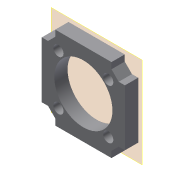
# Autodesk Inventor part: 50_Cube_Insert_Thorlabs
Saved by Autodesk Inventor 2019.4 (Build 234330000, 330)
## iProperties
Created: 2019-07-01
Part Number: 50_Cube_Insert_Thorlabs
Material: Generic
Document SubType Name: Modeling
Designer: diederichbenedict
Density: 1 g/cm^3
Appearance: Default
Author: diederichbenedict
Autodesk Inventor part; units mm, degrees
ref_plane "YZ Plane" through (0, 0, 0) normal (1, 0, 0) x (0, 1, 0)
ref_plane "XZ Plane" through (0, 0, 0) normal (0, 1, 0) x (-1, 0, 0)
ref_plane "Work Plane1" through (0, 0, 10) normal (0, 0, 1) x (1, 0, 0)
sketch "Sketch1" plane through (0, 0, 10) normal (0, 0, 1) x (1, 0, 0)
  line L0 (-4.0299, -0.3538) -> (-2.2322, 1.4439) construction
  arc A0 (-1.4439, 2.2322) -> (-2.2322, 1.4439) centre (-0.9299, 0.9299) ccw construction
  line L1 (-1.4439, 2.2322) -> (0.3538, 4.0299) construction
  line L2 (-37.8299, 42.8299) -> (-37.8299, 37.8299) construction
  line L3 (-37.8299, 37.8299) -> (-42.9208, 37.8299) construction
  line L4 (-37.8299, 42.2137) -> (-37.8299, 45.8299) construction
  line L5 (-37.8299, 45.8299) -> (-4.0299, 45.8299) construction
  line L6 (-4.0299, 45.8299) -> (-4.0299, 42.2137) construction
  line L7 (-4.0299, 4.0299) -> (0.3538, 4.0299) projected
  circle A1 centre (-20.9299, 20.9299) radius 17.5 projected
  line L8 (-20.9299, 58.9723) -> (17.1124, 20.9299) construction
  line L9 (17.1124, 20.9299) -> (-20.9299, -17.1124) construction
  line L10 (-20.9299, -17.1124) -> (-58.9723, 20.9299) construction
  line L11 (-58.9723, 20.9299) -> (-20.9299, 58.9723) construction
  line L12 (-20.9299, 58.9723) -> (-20.9299, -17.1124) construction
  line L13 (17.1124, 20.9299) -> (-58.9723, 20.9299) construction
  line L14 (-20.9299, 58.9723) -> (32.8701, 58.9723) construction
  line L15 (-43.4299, 43.4299) -> (1.5701, 43.4299) construction
  line L16 (1.5701, 43.4299) -> (1.5701, -1.5701) construction
  line L17 (1.5701, -1.5701) -> (-43.4299, -1.5701) construction
  line L18 (-43.4299, -1.5701) -> (-43.4299, 43.4299) construction
  line L19 (-43.4299, 43.4299) -> (1.5701, -1.5701) construction
  line L20 (1.5701, 43.4299) -> (-43.4299, -1.5701) construction
  line L21 (-43.4299, 5.3876) -> (-43.4299, 36.4723)
  line L22 (-43.4299, 36.4723) -> (-36.4723, 43.4299)
  line L23 (-36.4723, 43.4299) -> (-5.3876, 43.4299)
  line L24 (-5.3876, 43.4299) -> (1.5701, 36.4723)
  line L25 (1.5701, 36.4723) -> (1.5701, 5.3876)
  line L26 (1.5701, 5.3876) -> (-5.3876, -1.5701)
  line L27 (-5.3876, -1.5701) -> (-36.4723, -1.5701)
  line L28 (-36.4723, -1.5701) -> (-43.4299, 5.3876)
  line L29 (-4.0299, 42.2137) -> (-37.8299, 42.2137) projected
  line L30 (-4.0299, -0.3538) -> (-4.0299, 4.0299) projected
  point P0 (-37.8299, 4.0299)
  point P1 (-20.9299, 20.9299)
  dimension "d18" = 53.8
  dimension "d19" = 45
  dimension "d20" = 53.8
  dimension "d21" = 45
  dimension "d22" = 45
  constraints: 42 end point, 15 point on line, 5 midpoint, 4 parallel, 3 perpendicular, 2 horizontal, 1 equal length
  measures "d18" distance of L8.start L8.end
  measures "d19" angle of L8 L14
  measures "d20" distance of L8.end L9.end
  measures "d21" distance of L16.end L17.end
  measures "d22" distance of L15.end L16.end
extrude "Extrusion1" add sketch "Sketch1" along normal blind 8
sketch "Sketch2" plane through (0, 0, 18) normal (0, 0, 1) x (1, 0, 0)
  circle A0 centre (-35.9299, 35.9299) radius 3.0099 construction
  circle A1 centre (-5.93, 35.9299) radius 3.0099 construction
  circle A2 centre (-5.93, 5.93) radius 3.0099 construction
  circle A3 centre (-35.9299, 5.93) radius 3.0099 construction
  circle A4 centre (-35.9299, 35.9299) radius 3.05
  circle A5 centre (-5.93, 35.9299) radius 3.05
  circle A6 centre (-5.93, 5.93) radius 3.05
  circle A7 centre (-35.9299, 5.93) radius 3.05
  point P0 (0, 0)
  dimension "d30" = 6.1
  dimension "d31" = 6.1
  dimension "d32" = 6.1
  dimension "d33" = 6.1
  constraints: 4 centre point
  measures "d30" diameter of A4
  measures "d31" diameter of A5
  measures "d32" diameter of A6
  measures "d33" diameter of A7
ref_plane "Work Plane2" through (-40.9959, 0.8639, 22.2359) normal (0, 0, 1) x (1, 0, 0)
extrude "Extrusion2" cut sketch "Sketch2" against normal through all
sketch "Sketch3" plane through (0, 0, 10) normal (0, 0, -1) x (-1, 0, 0)
  line L0 (37.8299, -0.4701) -> (37.8299, 4.0299) construction
  line L1 (4.0299, 4.0299) -> (4.0299, -0.4701) construction
  line L2 (37.8299, -0.4701) -> (37.8299, 1.1886) construction
  line L3 (4.0299, -3.9701) -> (4.0299, -0.3538) construction
  line L4 (45.8299, 4.0299) -> (42.2137, 4.0299) construction
  line L5 (-0.3538, 4.0299) -> (-3.9701, 4.0299) construction
  line L6 (-3.9701, 37.8299) -> (-0.3538, 37.8299) construction
  line L7 (4.0299, 42.2137) -> (4.0299, 45.8299) construction
  line L8 (37.8299, 45.8299) -> (37.8299, 42.2137) construction
  line L9 (42.2137, 37.8299) -> (45.8299, 37.8299) construction
  line L10 (40.4657, 37.7299) -> (45.8299, 37.7299)
  line L11 (45.8299, 37.7299) -> (45.8299, 4.1299)
  line L12 (45.8299, 4.1299) -> (40.4657, 4.1299)
  line L13 (40.4657, 4.1299) -> (40.4657, 37.7299)
  line L14 (37.7299, 2.4952) -> (4.1299, 2.4952)
  line L15 (4.1299, 2.4952) -> (4.1299, -3.9701)
  line L16 (4.1299, -3.9701) -> (37.7299, -3.9701)
  line L17 (37.7299, -3.9701) -> (37.7299, 2.4952)
  line L18 (1.8946, 4.1299) -> (-3.9701, 4.1299)
  line L19 (-3.9701, 4.1299) -> (-3.9701, 37.7299)
  line L20 (-3.9701, 37.7299) -> (1.8946, 37.7299)
  line L21 (1.8946, 37.7299) -> (1.8946, 4.1299)
  line L22 (4.1299, 40.7326) -> (37.7299, 40.7326)
  line L23 (37.7299, 40.7326) -> (37.7299, 45.8299)
  line L24 (37.7299, 45.8299) -> (4.1299, 45.8299)
  line L25 (4.1299, 45.8299) -> (4.1299, 40.7326)
  point P0 (0, 0)
  dimension "d23" = 0.1
  dimension "d24" = 0.1
  dimension "d25" = 0.1
  dimension "d26" = 0.1
  dimension "d27" = 0.1
  constraints: 32 end point, 8 parallel, 4 horizontal, 4 perpendicular, 3 point on line
  measures "d23" distance between parallel lines of L8 L23
  measures "d24" distance between parallel lines of L7 L25
  measures "d25" distance between parallel lines of L6 L20
  measures "d26" distance between parallel lines of L5 L18
  measures "d27" distance between parallel lines of L1 L15
extrude "Extrusion3" add sketch "Sketch3" against normal up to surface (8 mm away)
sketch "Sketch4" plane through (0, 0, 18) normal (0, 0, 1) x (1, 0, 0)
  line L0 (3.9701, 4.1299) -> (0.3124, 4.1299) projected
  line L1 (3.9701, 37.7299) -> (3.9701, 4.1299) projected
  line L2 (0.3124, 37.7299) -> (3.9701, 37.7299) projected
  line L3 (0.3124, 37.7299) -> (-4.1299, 42.1723) projected
  line L4 (-4.1299, 45.8299) -> (-4.1299, 42.1723) projected
  line L5 (-37.7299, 45.8299) -> (-4.1299, 45.8299) projected
  line L6 (-37.7299, 42.1723) -> (-37.7299, 45.8299) projected
  line L7 (-37.7299, 42.1723) -> (-42.1723, 37.7299) projected
  line L8 (-45.8299, 37.7299) -> (-42.1723, 37.7299) projected
  line L9 (-45.8299, 4.1299) -> (-45.8299, 37.7299) projected
  line L10 (-42.1723, 4.1299) -> (-45.8299, 4.1299) projected
  line L11 (-42.1723, 4.1299) -> (-37.7299, -0.3124) projected
  line L12 (-37.7299, -3.9701) -> (-37.7299, -0.3124) projected
  line L13 (-4.1299, -3.9701) -> (-37.7299, -3.9701) projected
  line L14 (-4.1299, -0.3124) -> (-4.1299, -3.9701) projected
  line L15 (-4.1299, -0.3124) -> (0.3124, 4.1299) projected
  circle A0 centre (-20.9299, 20.9299) radius 17.5 projected
  circle A1 centre (-35.9299, 5.93) radius 3.05 projected
  circle A2 centre (-5.93, 35.9299) radius 3.05 projected
  circle A3 centre (-35.9299, 35.9299) radius 3.05 projected
  circle A4 centre (-5.93, 5.93) radius 3.05 projected
  line L16 (-3.9799, 45.9799) -> (-3.9799, 42.2344)
  line L17 (-3.9799, 42.2344) -> (0.3745, 37.8799)
  line L18 (0.3745, 37.8799) -> (4.1201, 37.8799)
  line L19 (4.1201, 37.8799) -> (4.1201, 3.9799)
  line L20 (4.1201, 3.9799) -> (0.3745, 3.9799)
  line L21 (0.3745, 3.9799) -> (-3.9799, -0.3745)
  line L22 (-3.9799, -0.3745) -> (-3.9799, -4.1201)
  line L23 (-3.9799, -4.1201) -> (-37.8799, -4.1201)
  line L24 (-37.8799, -4.1201) -> (-37.8799, -0.3745)
  line L25 (-37.8799, -0.3745) -> (-42.2344, 3.9799)
  line L26 (-42.2344, 3.9799) -> (-45.9799, 3.9799)
  line L27 (-45.9799, 3.9799) -> (-45.9799, 37.8799)
  line L28 (-45.9799, 37.8799) -> (-42.2344, 37.8799)
  line L29 (-42.2344, 37.8799) -> (-37.8799, 42.2344)
  line L30 (-37.8799, 42.2344) -> (-37.8799, 45.9799)
  line L31 (-37.8799, 45.9799) -> (-3.9799, 45.9799)
  point P0 (0, 0)
  dimension "d34" = 0.15
  constraints: 32 end point, 15 other
  measures "d34" distance between parallel lines of L5 L31
extrude "Extrusion4" add sketch "Sketch4" against normal up to surface (8 mm away) contours L16 L17 L18 L19 L20 L21 L22 L23 L24 L25 L26 L27 L28 L29 L30 L31
body "Solid1"
